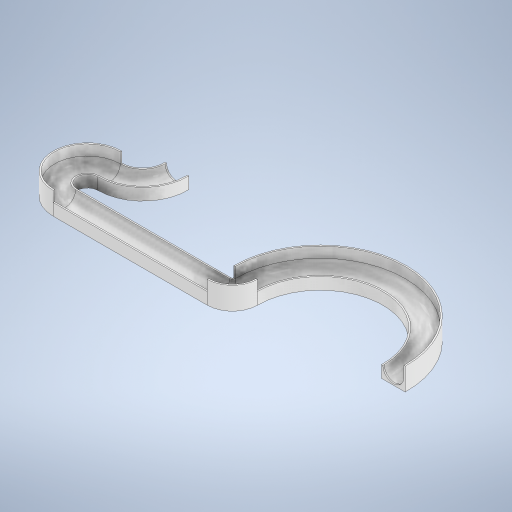
# Autodesk Inventor part: Agrupar bolinhas novamente
Saved by Autodesk Inventor 2024 (Build 280153000, 153)
## iProperties
Created: 2023-05-11
Part Number: Agrupar bolinhas novamente
Material: Plástico PET
Document SubType Name: Modeling
Designer: jpjoa
Density: 1.541 g/cm^3
Appearance: Branco
Author: jpjoa
Autodesk Inventor part; units mm, degrees
ref_plane "YZ Plane" through (0, 0, 0) normal (1, 0, 0) x (0, 1, 0)
ref_plane "XZ Plane" through (0, 0, 0) normal (0, 1, 0) x (-1, 0, 0)
ref_plane "XY Plane" through (0, 0, 0) normal (0, 0, 1) x (1, 0, 0)
sketch "Esboço1" plane through (0, 0, 0) normal (0, 1, 0) x (-1, 0, 0)
  arc A0 (-292.0445, -21.6) -> (-182.0445, -21.6) centre (-237.0445, -21.6) ccw
  line L0 (-292.0445, -21.6) -> (-237.0445, -21.6) construction
  line L1 (-182.0445, -21.6) -> (-237.0445, -21.6) construction
  arc A1 (-161.6445, -1.2) -> (-182.0445, -21.6) centre (-161.6445, -21.6) ccw
  line L2 (-182.0445, -21.6) -> (-161.6445, -21.6) construction
  line L3 (-161.6445, -1.2) -> (-161.6445, -21.6) construction
  arc A2 (-29.4, -57.6) -> (-29.4, -1.2) centre (-29.4, -29.4) ccw
  line L4 (-29.4, -1.2) -> (-29.4, -29.4) construction
  line L5 (-29.4, -57.6) -> (-29.4, -29.4) construction
  arc A3 (-29.4, -57.6) -> (-48.64, -76.8399) centre (-29.4, -76.8399) ccw
  line L6 (-29.4, -57.6) -> (-29.4, -76.8399) construction
  line L7 (-48.64, -76.8399) -> (-29.4, -76.8399) construction
  line L8 (-29.4, -1.2) -> (-161.6445, -1.2)
  arc A4 (-310.0445, -21.6) -> (-164.0445, -21.6) centre (-237.0445, -21.6) ccw
  arc A5 (-161.6445, -19.2) -> (-164.0445, -21.6) centre (-161.6445, -21.6) ccw
  line L9 (-161.6445, -19.2) -> (-29.4, -19.2)
  arc A6 (-29.4, -39.6) -> (-29.4, -19.2) centre (-29.4, -29.4) ccw
  arc A7 (-29.4, -39.6) -> (-66.64, -76.8399) centre (-29.4, -76.8399) ccw
  line L10 (-48.64, -76.8399) -> (-66.64, -76.8399)
  line L11 (-292.0445, -21.6) -> (-310.0445, -21.6)
  arc A8 (-311.2348, -20.4) -> (-162.8445, -21.6) centre (-237.0445, -21.6) ccw
  line L12 (-311.2348, -20.4) -> (-290.8311, -20.4)
  arc A9 (-290.8311, -20.4) -> (-183.2445, -21.6) centre (-237.0445, -21.6) ccw
  arc A10 (-161.6445, 0) -> (-183.2445, -21.6) centre (-161.6445, -21.6) ccw
  line L13 (-161.6445, 0) -> (-29.4, 0)
  arc A11 (-29.4, -58.8) -> (-29.4, 0) centre (-29.4, -29.4) ccw
  arc A12 (-29.4, -58.8) -> (-47.4, -78.0399) centre (-29.4, -76.8399) ccw
  line L14 (-47.4, -78.0399) -> (-67.8212, -78.0399)
  arc A13 (-29.4, -38.4) -> (-67.8212, -78.0399) centre (-29.4, -76.8399) ccw
  arc A14 (-29.4, -38.4) -> (-29.4, -20.4) centre (-29.4, -29.4) ccw
  line L15 (-29.4, -20.4) -> (-161.6445, -20.4)
  arc A15 (-161.6445, -20.4) -> (-162.8445, -21.6) centre (-161.6445, -21.6) ccw
  line L16 (-66.64, -76.8399) -> (-66.64, -78.0399)
  line L17 (-48.64, -78.0399) -> (-48.64, -76.8399)
  line L18 (-310.0445, -21.6) -> (-310.0445, -20.4)
  line L19 (-292.0445, -21.6) -> (-292.0445, -20.4)
  line L20 (-164.0445, -21.6) -> (-162.8445, -21.6)
  line L21 (-182.0445, -21.6) -> (-183.2445, -21.6)
  line L22 (-161.6445, -1.2) -> (-161.6445, 0)
  line L23 (-161.6445, -20.4) -> (-161.6445, -19.2)
  line L24 (-29.4, -38.4) -> (-29.4, -39.6)
  line L25 (-29.4, -57.6) -> (-29.4, -58.8)
  line L26 (-29.4, -1.2) -> (-29.4, 0)
  point P0 (0, 0)
  point P1 (-163.4445, -21.6)
  point P2 (-95.5222, 0)
  point P3 (0, -29.4)
  point P4 (-95.5222, -20.4)
  point P5 (-301.0329, -20.4)
  point P6 (-161.6445, -0.6)
  point P7 (-182.6445, -21.6)
  point P8 (-161.6445, -19.8)
  point P9 (-183.2445, -21.6)
  point P10 (-182.0445, -21.6)
  point P11 (-164.0445, -21.6)
  point P12 (-162.8445, -21.6)
  point P13 (-29.4, -39)
  point P14 (-29.4, -58.2)
  point P15 (-29.4, -0.6)
  point P16 (-29.4, -58.8)
  point P17 (-29.4, -57.6)
  point P18 (-29.4, -1.2)
  point P19 (-29.4, 0)
  dimension "d22" = 180
  dimension "d23" = 110
  dimension "d24" = 90
  dimension "d25" = 180
  dimension "d26" = 90
  dimension "d27" = 18
  dimension "d28" = 18
  dimension "d29" = 18
  dimension "d30" = 20.4
  dimension "d31" = 1.2
  dimension "d32" = 18
  dimension "d33" = 132.2445
  constraints: 54 end point, 47 point on circle, 16 centre point, 12 vertical alignment, 10 midpoint, 9 horizontal alignment, 4 perpendicular, 4 point on line, 2 horizontal, 2 parallel, 2 tangent, 13 other
  measures "d22" angle of L0 L1
  measures "d23" distance of L0.start L1.start
  measures "d24" angle of L3 L2
  measures "d25" angle of L4 L5
  measures "d26" angle of L6 L7
  measures "d27" radial gap between concentric circles of A0 A4
  measures "d28" radial gap between concentric circles of A2 A6
  measures "d29" radial gap between concentric circles of A3 A7
  measures "d30" distance of A6.start L9.end
  measures "d31" radial gap between concentric circles of A4 A8
  measures "d32" horizontal distance of L14.start L4.end
  measures "d33" distance of L13.start L13.end
extrude "Extrusão1" add sketch "Esboço1" against normal blind 1.2
extrude "Extrusão2" add sketch "Esboço1" along normal blind 9 contours L19 L12 A9 L21 A0 | L22 L13 L26 L8 | A5 L23 A15 L20 | L9 A6 L24 A14 L15 L23 | L25 A12 L14 L17 A3 | A7 L16 L14 A13 L24
extrude "Extrusão3" add sketch "Esboço1" along normal blind 18 contours L21 A10 L22 A1 | A4 L20 A8 L12 L18 | L26 A11 L25 A2
fillet "Arredondamento1" radius 9 14 edges at (95.5222, 0, -1.2) (176.0695, 0, -7.175) (237.0445, 0, -76.6) (292.0445, 0, -21) (43.0047, 0, -63.2352) (48.64, 0, -77.4399) (1.2, 0, -29.4) (19.2, 0, -29.4) (55.7326, 0, -50.5073) (66.64, 0, -77.4399) (163.3415, 0, -19.9029) (237.0445, 0, -94.6) (310.0445, 0, -21) (95.5222, 0, -19.2)
equation "\"d27\" = Diâmetro_esfera"
equation "\"d28\" = Diâmetro_esfera"
equation "\"d29\" = Diâmetro_esfera"
equation "\"Diâmetro_esfera\" = 18"
equation "\"Filamento\" = 0.4"
equation "\"Margem\" = 3 * Filamento"
equation "\"Parafuso\" = 3"
